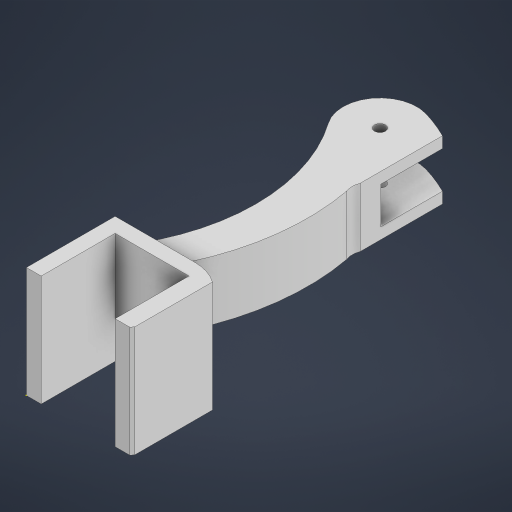
# Autodesk Inventor part: shok_absorber_holder
Saved by Autodesk Inventor 2024 (Build 280153000, 153)
## iProperties
Created: 2023-10-12
Part Number: shok_absorber_holder
Material: Типовые
Document SubType Name: Modeling
Designer: user
Density: 1 g/cm^3
Appearance: По умолчанию
Mass: 80.4086 g
Surface Area: 154.626 cm^2
Volume: 80.4086 cm^3
Author: user
Autodesk Inventor part; units mm, degrees
ref_plane "YZ Plane" through (0, 0, 0) normal (1, 0, 0) x (0, 1, 0)
sketch "Эскиз1" plane through (0, 0, 0) normal (0, 0, 1) x (1, 0, 0)
  line L0 (0, 0) -> (20, 0) construction
  line L1 (20, 0) -> (20, 20) construction
  line L2 (20, 20) -> (0, 20) construction
  line L3 (0, 20) -> (0, 0) construction
  line L4 (0, 0) -> (0, 20)
  line L5 (0, 0) -> (-4, 0)
  line L6 (-4, 0) -> (-4, 24)
  line L7 (-4, 24) -> (24, 24)
  line L8 (24, 24) -> (24, 0)
  line L9 (24, 0) -> (20, 0)
  line L10 (20, 0) -> (20, 20)
  line L11 (20, 20) -> (0, 20)
  dimension "d0" = 20
  dimension "d1" = 4
  dimension "d2" = 4
  constraints: 24 end point, 6 perpendicular, 5 equal length, 2 horizontal, 1 point on line, 1 vertical
  measures "d0" distance of L1.end L2.end
  measures "d1" distance of L8.end L0.end
  measures "d2" horizontal distance of L7.end L1.end
extrude "Выдавливание1" add sketch "Эскиз1" along normal blind 30
sketch "Эскиз2" plane through (0, 0, 30) normal (0, 0, 1) x (1, 0, 0)
  line L0 (24, 0) -> (24, 24) projected
  arc A0 (24, 0) -> (38.6, 61.3222) centre (-41.6488, 48.0293) ccw
  arc A1 (38.6, 61.3222) -> (7.0088, 97.1053) centre (-5.7899, 53.9692) ccw
  line L1 (-4, 24) -> (-4, 0) projected
  arc A2 (-4, 24) -> (-4, 81.744) centre (-44.8217, 52.872) ccw
  arc A3 (7.0088, 97.1053) -> (-4, 81.744) centre (4.1643, 87.5184) ccw
  circle A4 centre (4.1643, 87.5184) radius 1.5
  line L2 (24, 24) -> (-4, 24) projected
  point P0 (0, 0)
  dimension "d5" = 10
  dimension "d6" = 3
  dimension "d7" = 50
  constraints: 8 point on circle, 5 centre point, 3 tangent, 1 coincident, 1 vertical alignment
  measures "d5" radius of A3
  measures "d6" diameter of A4
  measures "d7" radius of A2
extrude "Выдавливание2" add sketch "Эскиз2" against normal up to surface (30 mm away)
ref_plane "РабПлоскость1" through (-5.8357, 87.5184, 30) normal (-1, 0, 0) x (0, 0, 1)
sketch "Эскиз4" plane through (-5.8357, 87.5184, 30) normal (-1, 0, 0) x (0, 0, 1)
  line L0 (-20, 10) -> (-10, 10)
  line L1 (-10, 10) -> (-10, -10)
  line L2 (-10, -10) -> (-20, -10)
  line L3 (-20, -10) -> (-20, 10)
  line L4 (0, 10) -> (-30, 10) projected
  point P0 (-30, -87.5184)
  point P1 (-15, 10)
  dimension "d10" = 10
  dimension "d11" = 20
  constraints: 8 end point, 2 midpoint, 2 parallel, 1 horizontal, 1 perpendicular
  measures "d10" distance between parallel lines of L3 L1
  measures "d11" distance of L0.end L1.end
extrude "Выдавливание3" cut sketch "Эскиз4" against normal through all
sketch "Эскиз5" plane through (-5.8357, 87.5184, 30) normal (-1, 0, 0) x (0, 0, 1)
  line L0 (-30, -26.1962) -> (-30, -87.5184) projected
  line L1 (-30, -63.5184) -> (-23, -63.5184)
  line L2 (-23, -63.5184) -> (-23, -16.5184)
  line L3 (-23, -16.5184) -> (-30, -16.5184)
  line L4 (-30, -16.5184) -> (-30, -63.5184)
  line L5 (-30, -63.5184) -> (0, -63.5184) projected
  dimension "d14" = 7
  dimension "d15" = 47
  constraints: 8 end point, 2 parallel, 2 point on line, 1 horizontal, 1 perpendicular
  measures "d14" distance of L2.end L3.end
  measures "d15" distance of L3.end L1.start
extrude "Выдавливание4" cut sketch "Эскиз5" against normal through all
ref_plane "РабПлоскость2" through (0, 0, 15) normal (0, 0, -1) x (-1, 0, 0)
mirror "Зеркальное отражение1" about plane through (0, 0, 15) normal (0, 0, -1) of "Выдавливание4"
fillet "Сопряжение1" radius 12 2 edges at (36.0633, 24, 3.5) (36.0633, 24, 26.5)
fillet "Сопряжение2" radius 12 2 edges at (35.8572, 71, 3.5) (35.8572, 71, 26.5)
sketch "Эскиз6" plane through (-4, 24, 23) normal (0, 0, 1) x (1, 0, 0)
  arc A0 (17, 4.7391) -> (22, 45) centre (-43.2292, 32.6599) ccw construction
  arc A1 (20.3144, 3.2026) -> (25.5896, 45.6791) centre (-43.2292, 32.6599) ccw
  arc A2 (13.6856, 6.2756) -> (18.4104, 44.3209) centre (-43.2292, 32.6599) ccw
  arc A3 (13.6856, 6.2756) -> (20.3144, 3.2026) centre (17, 4.7391) ccw
  arc A4 (25.5896, 45.6791) -> (18.4104, 44.3209) centre (22, 45) ccw
  line L0 (0, 0) -> (0, -24) projected
  point P0 (4, -24)
  dimension "d20" = 17
  dimension "d21" = 45
  dimension "d22" = 22
  constraints: 10 point on circle, 5 centre point, 4 tangent
  measures "d20" distance from line of L0 A0.start
  measures "d21" vertical distance of L0.start A0.end
  measures "d22" distance from line of L0 A0.end
extrude "Выдавливание5" cut sketch "Эскиз6" against normal through all
sketch "Эскиз7" plane through (-4, 24, 23) normal (0, 0, 1) x (1, 0, 0)
  arc A0 (31.8516, -18.235) -> (42.6, 37.3222) centre (-37.6488, 24.0293) ccw projected
  arc A1 (31.8516, -18.235) -> (21.5986, 0) centre (21.5986, -12) ccw projected
  arc A2 (42.6, 37.3222) -> (19.593, 69.5583) centre (-1.7899, 29.9692) ccw projected
  arc A3 (13.8903, 47) -> (19.593, 69.5583) centre (13.8903, 59) ccw projected
  arc A4 (13.6856, 6.2756) -> (18.4104, 44.3209) centre (-43.2292, 32.6599) ccw projected
  arc A5 (13.8903, 47) -> (19.593, 69.5583) centre (13.8903, 59) ccw projected
  arc A6 (18.4174, 47.8867) -> (19.593, 69.5583) centre (13.9238, 58.9982) ccw
  line L0 (0, 0) -> (21.5986, 0) projected
  arc A7 (13.9667, 6.8907) -> (21.5986, 0) centre (18.8905, 4.6723) ccw
  arc A8 (18.4174, 47.8867) -> (18.4104, 44.3209) centre (22.8221, 46.0952) ccw
  point P0 (4, -24)
  point P1 (19.6658, 69.519)
  point P2 (16.1824, 0)
  constraints: 8 point on circle, 3 centre point, 1 tangent
extrude "Выдавливание6" cut sketch "Эскиз7" against normal blind 36 contours A1 L0 A7 A4 A8 A6 A2 A0
sketch "Эскиз8" plane through (-4, 0, 0) normal (-1, 0, 0) x (0, 0, 1)
  point P0 (0, 0)
sketch "Эскиз9" plane through (-5.8357, 87.5184, 30) normal (-1, 0, 0) x (0, 0, 1)
  line L0 (-23, -16.5184) -> (-23, -63.5184) projected
  line L1 (-23, -16.5184) -> (-46.8016, -16.5184)
  line L2 (-46.8016, -16.5184) -> (-46.8016, 17.3569)
  line L3 (-46.8016, 17.3569) -> (-23, 17.3569)
  line L4 (-23, 17.3569) -> (-23, -16.5184)
  point P0 (-30, -87.5184)
  constraints: 8 end point, 2 parallel, 1 horizontal, 1 perpendicular
extrude "Выдавливание7" cut sketch "Эскиз9" against normal blind 36
mirror "Зеркальное отражение2" about plane through (0, 0, 15) normal (0, 0, -1) of "Выдавливание7"
sketch "Эскиз10" plane through (0, 0, 30) normal (0, 0, 1) x (1, 0, 0)
  line L0 (24.5745, 0) -> (35.4567, 0)
  line L1 (35.4567, 0) -> (35.4567, 28.8198)
  line L2 (35.4567, 28.8198) -> (24.5745, 28.8198)
  line L3 (24.5745, 28.8198) -> (24.5745, 0)
  point P0 (0, 0)
  constraints: 8 end point, 2 parallel, 1 horizontal, 1 perpendicular
extrude "Выдавливание8" cut sketch "Эскиз10" against normal through all
sketch "Эскиз11" plane through (-44.8217, 52.872, 23) normal (0, 0, 1) x (1, 0, 0)
  arc A0 (59.2391, 19.0147) -> (60.4874, 40.647) centre (54.7454, 30.1262) ccw projected
  line L0 (59.2391, 19.0147) -> (70.8374, 19.0147)
  line L1 (70.8374, 19.0147) -> (70.8374, 43.6051)
  line L2 (70.8374, 43.6051) -> (59.2391, 43.6051)
  line L3 (59.2391, 43.6051) -> (59.2391, 19.0147)
  point P0 (44.8217, -52.872)
  constraints: 8 end point, 2 parallel, 1 horizontal, 1 perpendicular
extrude "Выдавливание9" cut sketch "Эскиз11" against normal through all
